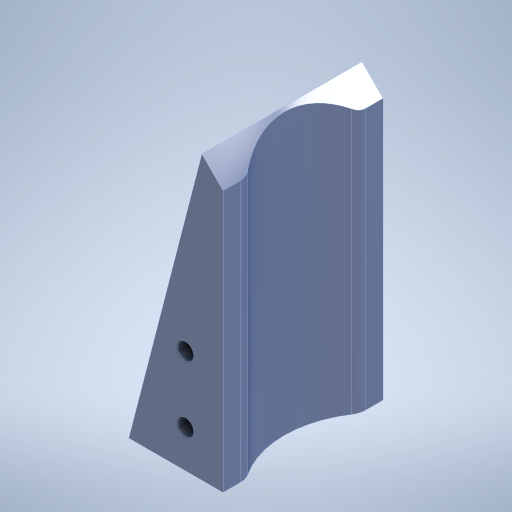
# Autodesk Inventor part: Gripper
Saved by Autodesk Inventor 2024.2 (Build 282272000, 272)
## iProperties
Created: 2025-03-19
Part Number: Gripper
Material: Generic
Document SubType Name: Modeling
Designer: migue
Density: 1 g/cm^3
Appearance: Flaked Satin - Blue
Author: migue
Autodesk Inventor part; units mm, degrees
ref_plane "YZ Plane" through (0, 0, 0) normal (1, 0, 0) x (0, 1, 0)
ref_plane "XZ Plane" through (0, 0, 0) normal (0, 1, 0) x (-1, 0, 0)
sketch "Sketch1" plane through (0, 0, 0) normal (0, 1, 0) x (-1, 0, 0)
  line L0 (0, 0) -> (-20, 0)
  line L1 (-20, 0) -> (-20, -34)
  line L2 (-20, -34) -> (0, -34)
  line L3 (0, -34) -> (0, 0)
  dimension "d0" = 34
  dimension "d1" = 20
  constraints: 8 end point, 2 parallel, 1 horizontal, 1 perpendicular
  measures "d0" distance of L2.end L0.start
  measures "d1" distance of L0.start L0.end
extrude "Extrusion1" add sketch "Sketch1" along normal blind 60
chamfer "Chamfer1" distance 4.5 angle 45 1 edges at (20, 60, -17)
sketch "Sketch3" plane through (0, 0, 0) normal (0, 0, 1) x (1, 0, 0)
  line L0 (0, 60) -> (15.5, 60) projected
  line L1 (15.5, 60) -> (0, 0)
  line L2 (0, 0) -> (20, 0) projected
  line L3 (20, 0) -> (0, 0)
  line L4 (0, 0) -> (0, 60)
  line L5 (0, 60) -> (20, 60)
  line L6 (20, 60) -> (20, 0)
  constraints: 10 end point, 2 parallel, 1 horizontal, 1 perpendicular
extrude "Extrusion2" cut sketch "Sketch3" against normal blind 60 contours L0 L1 L4
sketch "Sketch8" plane through (0, 0, 0) normal (0, -1, 0) x (1, 0, 0)
  line L0 (20, 0) -> (20, -34) projected
  line L1 (20, -17) -> (36, -17) construction
  circle A0 centre (36, -17) radius 20
  point P0 (0, 0)
  point P1 (20, -29)
  point P2 (20, -5)
  dimension "d44" = 40
  dimension "d45" = 16
  constraints: 2 end point, 1 centre point, 1 coincident, 1 horizontal, 1 midpoint
  measures "d44" diameter of A0
  measures "d45" distance of L1.start L1.end
extrude "Extrusion7" cut sketch "Sketch8" against normal through all contours L0 A0 picked at (19.2708, -19.7731)
shell "Shell2" thickness 3 removed faces 1 at (10.3333, 40, -22.6667)
sketch "Sketch9" plane through (0, 0, 0) normal (0, -1, 0) x (1, 0, 0)
  circle A0 centre (5, -4.5) radius 2.25
  line L0 (0, 0) -> (20, 0) projected
  line L1 (0, -34) -> (0, 0) projected
  line L2 (5, -4.5) -> (15, -4.5) construction
  line L3 (14.629, -8.4982) -> (14.629, -3) projected
  line L4 (5, -4.5) -> (15, -4.5) construction
  circle A1 centre (15, -4.5) radius 2.25
  line L5 (0, -17) -> (10, -17) construction
  circle A2 centre (5, -29.5) radius 2.25
  circle A3 centre (15, -29.5) radius 2.25
  dimension "d49" = 4.5
  dimension "d50" = 4.5
  dimension "d51" = 5
  dimension "d52" = 10
  dimension "d53" = 360
  dimension "d54" = 4.5
  dimension "d56" = 25
  constraints: 6 end point, 4 centre point, 2 horizontal, 2 symmetric about line, 1 coincident, 1 collinear, 1 midpoint, 1 perpendicular, 2 other
  measures "d49" diameter of A0
  measures "d50" distance from line of L2.start L0
  measures "d51" distance from line of L1 L2.start
  measures "d52" distance of L2.start L2.end
  measures "d54" diameter of A1
  measures "d56" distance of A3.centre L2.end
extrude "Extrusion8" cut sketch "Sketch9" against normal blind 3
fillet "Fillet2" radius 4 2 edges at (20, 27.75, -5) (20, 27.75, -29)
sketch "Sketch10" plane through (20, 0, 0) normal (0, 0, 1) x (1, 0, 0)
  circle A0 centre (-8, 8) radius 1.75
  line L0 (-8, 8) -> (-8, 22) construction
  circle A1 centre (-8, 22) radius 1.75
  point P0 (-20, 0)
  dimension "d60" = 3.5
  dimension "d61" = 12
  dimension "d62" = 8
  dimension "d64" = 3.5
  constraints: 2 centre point, 2 end point, 1 coincident, 1 vertical
  measures "d60" diameter of A0
  measures "d61" horizontal distance of point (-20, 0) L0.start
  measures "d62" vertical distance of point (-20, 0) L0.start
  measures "d64" diameter of A1
extrude "Extrusion9" cut sketch "Sketch10" against normal blind 3
ref_plane "Work Plane1" through (0, 0, -17) normal (0, 0, 1) x (1, 0, 0)
mirror "Mirror1" about plane through (0, 0, -17) normal (0, 0, 1) of "Extrusion9"
body "Solid1"
